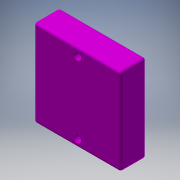
# Autodesk Inventor part: calle-patin
Saved by Autodesk Inventor 2017 (Build 210142000, 142)
## iProperties
Created: 2018-04-14
Part Number: calle-patin
Material: Generic
Document SubType Name: Modeling
Designer: franc
Density: 1 g/cm^3
Appearance: Default
Author: franc
Autodesk Inventor part; units mm, degrees
ref_plane "YZ Plane" through (0, 0, 0) normal (1, 0, 0) x (0, 1, 0)
ref_plane "XZ Plane" through (0, 0, 0) normal (0, 1, 0) x (-1, 0, 0)
ref_plane "XY Plane" through (0, 0, 0) normal (0, 0, 1) x (1, 0, 0)
sketch "Esquisse1" plane through (0, 0, 0) normal (0, 1, 0) x (-1, 0, 0)
  line L0 (7.7669, 22.1799) -> (-26.2331, 22.1799)
  line L1 (-26.2331, 22.1799) -> (-26.2331, -11.8201)
  line L2 (-26.2331, -11.8201) -> (7.7669, -11.8201)
  line L3 (7.7669, -11.8201) -> (7.7669, 22.1799)
  point P0 (0, 0)
  dimension "d0" = 34
  dimension "d1" = 34
  constraints: 8 end point, 2 parallel, 1 horizontal, 1 perpendicular
  measures "d0" distance of L2.end L1.end
  measures "d1" distance of L2.end L0.start
extrude "Extrusion1" add sketch "Esquisse1" along normal blind 10
sketch "Esquisse2" plane through (0, 10, 0) normal (0, 1, 0) x (1, 0, 0)
  circle A0 centre (-2.7669, -17.1799) radius 1.5
  circle A1 centre (21.2331, 6.8201) radius 1.5
  line L0 (-7.7669, 11.8201) -> (-7.7669, -22.1799) projected
  line L1 (-7.7669, -22.1799) -> (26.2331, -22.1799) projected
  line L2 (26.2331, 11.8201) -> (-7.7669, 11.8201) projected
  line L3 (26.2331, -22.1799) -> (26.2331, 11.8201) projected
  point P0 (0, 0)
  dimension "d4" = 3
  dimension "d5" = 3
  dimension "d6" = 5
  dimension "d8" = 5
  dimension "d9" = 5
  dimension "d13" = 5
  constraints: 2 centre point
  measures "d4" diameter of A0
  measures "d5" diameter of A1
  measures "d6" distance from line of L0 A0.centre
  measures "d8" distance from line of L1 A0.centre
  measures "d9" distance from line of L2 A1.centre
  measures "d13" distance from line of L3 A1.centre
extrude "Extrusion2" cut sketch "Esquisse2" against normal blind 10 contours A0 | A1
fillet "Congé1" radius 1 12 edges at (9.2331, 10, 22.1799) (26.2331, 10, 5.1799) (9.2331, 10, -11.8201) (-7.7669, 10, 5.1799) (-7.7669, 0, 5.1799) (9.2331, 0, -11.8201) (26.2331, 0, 5.1799) (9.2331, 0, 22.1799) (26.2331, 5, 22.1799) (26.2331, 5, -11.8201) (-7.7669, 5, -11.8201) (-7.7669, 5, 22.1799)
